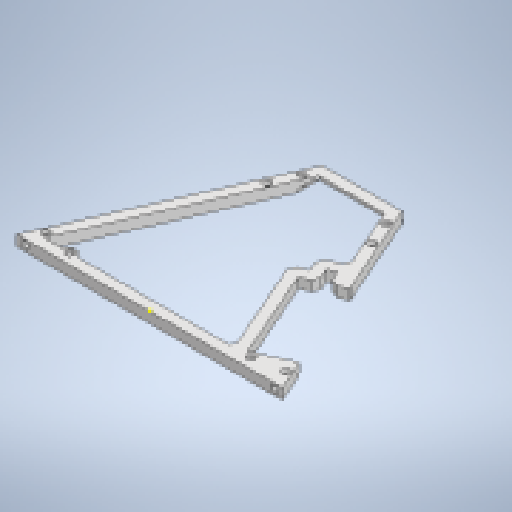
# Autodesk Inventor part: BottomPlate
Saved by Autodesk Inventor 2025.2 (Build 292293000, 293)
## iProperties
Created: 2025-08-10
Part Number: BottomPlate
Material: Generic
Document SubType Name: Modeling
Designer: hofma
Density: 1 g/cm^3
Appearance: Default
Author: hofma
Autodesk Inventor part; units mm, degrees
ref_plane "YZ Plane" through (0, 0, 0) normal (1, 0, 0) x (0, 1, 0)
ref_plane "XZ Plane" through (0, 0, 0) normal (0, 1, 0) x (-1, 0, 0)
ref_plane "XY Plane" through (0, 0, 0) normal (0, 0, 1) x (1, 0, 0)
sketch "Sketch1" plane through (0, 0, 0) normal (0, 1, 0) x (-1, 0, 0)
  line L0 (125, 0) -> (-125, 0)
  line L1 (-125, 0) -> (-37.5, -200)
  line L2 (-37.5, -200) -> (37.5, -200)
  line L3 (37.5, -200) -> (125, 0)
  point P0 (0, 0)
  point P1 (0, 0)
  point P2 (0, -200)
  dimension "d0" = 250
  dimension "d3" = 200
  dimension "d4" = 75
  constraints: 8 end point, 2 midpoint, 1 coincident, 1 horizontal, 1 parallel, 1 vertical alignment
  measures "d0" distance of L0.start L0.end
  measures "d3" distance between parallel lines of L2 L0
  measures "d4" distance of L1.end L2.end
extrude "Extrusion1" add sketch "Sketch1" along normal blind 10
sketch "Sketch2" plane through (37.5, 0, -200) normal (0, 0, -1) x (-1, 0, 0)
  line L0 (0, 0) -> (75, 0) projected
  line L1 (0, 0) -> (75, 0)
  line L2 (75, 0) -> (75, 7)
  line L3 (75, 7) -> (0, 7)
  line L4 (0, 7) -> (0, 0)
  line L5 (0, 10) -> (75, 10) projected
  point P0 (37.5, 7)
  point P1 (37.5, 0)
  dimension "d5" = 3
  dimension "d6" = 75
  constraints: 8 end point, 2 midpoint, 2 parallel, 1 horizontal, 1 perpendicular, 1 point on line, 1 vertical alignment
  measures "d5" distance between parallel lines of L3 L5
  measures "d6" distance of L2.end L3.end
extrude "Extrusion2" cut sketch "Sketch2" against normal blind 77
fillet "Fillet1" radius 7 2 edges at (37.5, 7, -161.5) (-37.5, 7, -161.5)
sketch "Sketch3" plane through (125, 0, 0) normal (0.9161573, 0, -0.4008188) x (-0.4008188, 0, -0.9161573)
  line L0 (30, -1.8) -> (31, 10)
  line L1 (100.2047, 10) -> (0, 10) projected
  line L2 (31, 10) -> (122.8, 10)
  line L3 (0, 10) -> (218.3031, 10) projected
  line L4 (122.8, 10) -> (123.8, -1.8)
  line L5 (30, -1.8) -> (123.8, -1.8)
  line L6 (0, 0) -> (0, 10) projected
  point P0 (50.1024, 0)
  point P1 (100.2047, 0)
  dimension "d10" = 1
  dimension "d11" = 1
  dimension "d12" = 93.8
  dimension "d16" = 11.8
  dimension "d17" = 30
  constraints: 8 end point, 2 point on line, 1 horizontal
  measures "d10" horizontal distance of L0.end L0.start
  measures "d11" horizontal distance of L4.end L2.end
  measures "d12" distance of L4.end L0.start
  measures "d16" distance between parallel lines of L5 L1
  measures "d17" distance from line of L6 L0.start
extrude "Extrusion3" cut sketch "Sketch3" against normal blind 37
sketch "Sketch4" plane through (0, 10, 0) normal (0, 1, 0) x (1, 0, 0)
  line L0 (41.8816, 97.6738) -> (75.7794, 112.5041) construction
  line L1 (55.1659, 103.4857) -> (49.1536, 117.2281)
  line L2 (49.1536, 117.2281) -> (56.4829, 120.4346)
  line L3 (56.4829, 120.4346) -> (62.4952, 106.6922)
  line L4 (62.4952, 106.6922) -> (55.1659, 103.4857)
  point P0 (0, 0)
  point P1 (58.8305, 105.089)
  dimension "d18" = 8
  dimension "d19" = 15
  constraints: 8 end point, 4 perpendicular, 2 midpoint, 1 point on line
  measures "d18" distance between parallel lines of L3 L1
  measures "d19" distance from line of L1.start L2
extrude "Extrusion4" cut sketch "Sketch4" against normal through all
sketch "Sketch5" plane through (0, 10, 0) normal (0, 1, 0) x (1, 0, 0)
  line L0 (56.4829, 120.4346) -> (62.4952, 106.6922) projected
  line L1 (62.4952, 106.6922) -> (75.7794, 112.5041) projected
  line L2 (75.7794, 112.5041) -> (37.5, 200) projected
  line L3 (37.5, 200) -> (-37.5, 200) projected
  line L4 (-37.5, 200) -> (-125, 0) projected
  line L5 (-125, 0) -> (125, 0) projected
  line L6 (125, 0) -> (112.5746, 28.4009) projected
  line L7 (112.5746, 28.4009) -> (78.6768, 13.5706) projected
  line L8 (78.6768, 13.5706) -> (41.8816, 97.6738) projected
  line L9 (41.8816, 97.6738) -> (55.1659, 103.4857) projected
  line L10 (55.1659, 103.4857) -> (49.1536, 117.2281) projected
  line L11 (49.1536, 117.2281) -> (56.4829, 120.4346) projected
  line L12 (-109.7098, 10) -> (-30.9598, 190)
  line L13 (-30.9598, 190) -> (30.9598, 190)
  line L14 (30.9598, 190) -> (56.5974, 131.3999)
  line L15 (56.5974, 131.3999) -> (35.9839, 122.3814)
  line L16 (35.9839, 122.3814) -> (41.9961, 108.6391)
  line L17 (41.9961, 108.6391) -> (28.7119, 102.8272)
  line L18 (28.7119, 102.8272) -> (73.5234, 0.4008)
  line L19 (73.5234, 0.4008) -> (95.4644, 10)
  line L20 (95.4644, 10) -> (-109.7098, 10)
  point P0 (0, 0)
  point P1 (69.3238, 10)
  dimension "d22" = 10
  constraints: 18 end point, 8 other
  measures "d22" distance between parallel lines of L4 L12
extrude "Extrusion5" cut sketch "Sketch5" against normal blind 10 contours L12 L13 L14 L15 L16 L17 L18 L20
sketch "Sketch10" plane through (0, 10, 0) normal (0, 1, 0) x (1, 0, 0)
  line L0 (-109.7098, 10) -> (69.3238, 10) projected
  line L1 (-87.5, 10) -> (-82.5, 10)
  line L2 (-82.5, 10) -> (-82.5, 15)
  line L3 (-82.5, 15) -> (-87.5, 15)
  line L4 (-87.5, 15) -> (-87.5, 10)
  line L5 (-125, 0) -> (125, 0) projected
  point P0 (0, 0)
  point P1 (0, 0)
  point P2 (-85, 15)
  point P3 (-82.5, 10)
  dimension "d52" = 5
  dimension "d53" = 85
  dimension "d54" = 5
  constraints: 8 end point, 2 midpoint, 2 parallel, 1 horizontal, 1 perpendicular, 1 point on line
  measures "d52" distance of L2.end L3.end
  measures "d53" horizontal distance of point (0, 0) point (-85, 15)
  measures "d54" distance between parallel lines of L0 L3
extrude "Extrusion6" add sketch "Sketch10" against normal up to surface (10 mm away)
sketch "Sketch6" plane through (-125, 0, 0) normal (0, 0, 1) x (1, 0, 0)
  line L0 (0, 0) -> (0, 10) projected
  line L1 (250, 0) -> (250, 10) projected
  point P0 (125, 0)
  point P1 (7.5, 5)
  point P2 (242.5, 5)
  point P3 (0, 5)
  dimension "d25" = 7.5
  dimension "d26" = 7.5
  constraints: 2 horizontal alignment, 1 midpoint
  measures "d25" distance from line of L0 point (7.5, 5)
  measures "d26" distance from line of L1 point (242.5, 5)
hole "Hole1" at (117.5, 5, 0) at (-117.5, 5, 0) direction (0, 0, -1) diameter 5.6 depth 8.1
sketch "Sketch7" plane through (0, 10, 0) normal (0, 1, 0) x (1, 0, 0)
  line L0 (0, 0) -> (0, -36.9997) construction
  line L1 (69.3238, 10) -> (-109.7098, 10) projected
  point P0 (-85, 10)
  point P1 (85, 10)
  dimension "d34" = 0
  dimension "d35" = 170
  constraints: 2 end point, 1 horizontal alignment, 1 symmetric about line, 1 vertical
  measures "d34" distance from line of L1 point (-85, 10)
  measures "d35" distance of point (85, 10) point (-85, 10)
hole "Hole2" at (-85, 10, -10) at (85, 10, -10) direction (0, -1, 0) diameter 5.6 depth 8.1
sketch "Sketch8" plane through (0, 10, 0) normal (0, 1, 0) x (1, 0, 0)
  line L0 (37.5, 200) -> (-37.5, 200) projected
  line L1 (0, 200) -> (0, 219.1453) construction
  line L2 (75.7794, 112.5041) -> (37.5, 200) projected
  point P0 (0, 0)
  point P1 (39.4799, 183)
  point P2 (-39.4799, 183)
  dimension "d43" = 5
  dimension "d44" = 17
  constraints: 2 end point, 1 midpoint, 1 symmetric about line, 1 vertical
  measures "d43" distance from line of L2 point (39.48, 183)
  measures "d44" distance from line of L0 point (39.48, 183)
hole "Hole3" at (39.4799, 10, -183) at (-39.4799, 10, -183) direction (0, -1, 0) diameter 5.6 depth 8.1
sketch "Sketch9" plane through (0, 10, 0) normal (0, 1, 0) x (1, 0, 0)
  point P0 (0, 0)
sketch "Sketch11" plane through (0, 10, 0) normal (0, 1, 0) x (1, 0, 0)
  line L0 (-119.6384, -0.2193) -> (-31.6935, 200.7975) construction
  line L1 (-37.5, 200) -> (-125, 0) projected
  line L2 (-37.5, 200) -> (-125, 0) projected
  line L3 (-125, 0) -> (125, 0) projected
  point P0 (0, 0)
  point P1 (-112.9799, 15)
  point P2 (-49.5424, 160)
  dimension "d57" = 5
  dimension "d58" = 15
  dimension "d59" = 160
  constraints: 2 end point, 2 parallel, 2 point on line
  measures "d57" distance between parallel lines of L1 L0
  measures "d58" distance from line of point (-112.98, 15) L3
  measures "d59" distance from line of point (-49.542, 160) L3
hole "Hole4" at (-112.9799, 10, -15) at (-49.5424, 10, -160) direction (0, -1, 0) diameter 4.5 end through all counterbore diameter 8 counterbore depth 4.6 clearance for "Socket Head Cap Screw ISO 4762" size "M4" standard "ISO"
mirror "Mirror1" about plane through (0, 0, 0) normal (1, 0, 0) of "Hole4"
chamfer "Chamfer1" distance 5 angle 45 5 edges at (28.7119, 5, -102.8272) (35.9839, 5, -122.3814) (54.9961, 5, -103.8739) (62.3253, 5, -107.0804) (56.5974, 5, -131.3999)
chamfer "Chamfer2" distance 5 angle 45 3 edges at (69.3238, 5, -10) (-82.5, 0.95, -10) (-87.5, 0.95, -10)
chamfer "Chamfer3" distance 1 angle 45 8 edges at (85, 10, -12.8) (39.4799, 10, -185.8) (-39.4799, 10, -185.8) (-82.2, 10, -10) (-49.5424, 0, -162.25) (-112.9799, 0, -17.25) (49.5424, 0, -162.25) (112.9799, 0, -17.25)
chamfer "Chamfer4" distance 1 angle 45 2 edges at (-117.5, 7.8, 0) (117.5, 7.8, 0)
chamfer "Chamfer5" distance 1 angle 45 2 edges at (112.7445, 5, -28.0127) (75.6096, 5, -112.8923)
chamfer "Chamfer6" distance 1 angle 45 3 edges at (0, 7, -200) (-35.4498, 4.9498, -200) (35.4498, 4.9498, -200)
equation "\"d26\" = d25"
body "Solid1"
